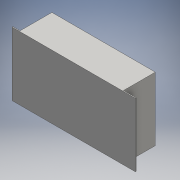
# Autodesk Inventor part: sound amplifier
Saved by Autodesk Inventor 2016 (Build 200138000, 138)
## iProperties
Created: 2017-06-06
Part Number: sound amplifier
Material: Generic
Document SubType Name: Modeling
Designer: fabio-note
Density: 1 g/cm^3
Appearance: Default
Author: fabio-note
Autodesk Inventor part; units mm, degrees
ref_plane "YZ Plane" through (0, 0, 0) normal (1, 0, 0) x (0, 1, 0)
ref_plane "XZ Plane" through (0, 0, 0) normal (0, 1, 0) x (-1, 0, 0)
ref_plane "XY Plane" through (0, 0, 0) normal (0, 0, 1) x (1, 0, 0)
sketch "Sketch1" plane through (0, 0, 0) normal (0, 1, 0) x (-1, 0, 0)
  line L0 (77.5, 40) -> (-77.5, 40)
  line L1 (-77.5, 40) -> (-77.5, -40)
  line L2 (-77.5, -40) -> (77.5, -40)
  line L3 (77.5, -40) -> (77.5, 40)
  point P0 (0, 0)
  point P1 (0, -40)
  point P2 (77.5, 0)
  dimension "d0" = 155
  dimension "d1" = 80
  constraints: 8 end point, 2 midpoint, 2 parallel, 1 horizontal, 1 horizontal alignment, 1 perpendicular, 1 vertical alignment
  measures "d0" distance of L1.end L2.end
  measures "d1" distance of L2.end L0.start
extrude "Extrusion1" add sketch "Sketch1" along normal blind 1
sketch "Sketch3" plane through (0, 1, 0) normal (0, 1, 0) x (1, 0, 0)
  line L0 (77.5, 40) -> (-77.5, 40) projected
  line L1 (-77.5, -40) -> (77.5, -40) projected
  line L2 (-68.3973, 40) -> (61.6027, 40)
  line L3 (61.6027, 40) -> (61.6027, -40)
  line L4 (61.6027, -40) -> (-68.3973, -40)
  line L5 (-68.3973, -40) -> (-68.3973, 40)
  point P0 (0, 0)
  point P1 (0, 40)
  dimension "d7" = 130
  constraints: 8 end point, 2 parallel, 2 point on line, 1 horizontal, 1 midpoint, 1 perpendicular, 1 vertical alignment
  measures "d7" distance between parallel lines of L3 L5
extrude "Extrusion2" add sketch "Sketch3" along normal blind 40
body "Solid1"
